Autodesk Inventor part; units mm, degrees
(part 2 of 2)
extrude "Выдавливание1" add sketch "Эскиз1" along normal blind 4 contours L16 L17 L18 L19 L20 L21 L22 L23 L24 L25 L26 L223
extrude "Выдавливание2" add sketch "Эскиз1" against normal blind 4 contours L214 A65 L215 L20 L19 L18 L17 L16 L15 | L15 L223 L27 L216 A66 L214 | L16 L17 L18 L19 L20 L21 L22 L23 L24 L25 L26 L223 | L26 L25 L24 L23 L22 L215 A64 L216 L27 | L217 L218 L219 L220 L221 L222
extrude "Выдавливание3" cut sketch "Эскиз1" against normal blind 4 contours L217 L218 L219 L220 L221 L222
extrude "Выдавливание4" add sketch "Эскиз1" against normal blind 2 contours L217 L218 L219 L220 L221 L222
